Autodesk Fusion 360 part; units mm, degrees
(part 3 of 5)
  constraint tangent L16 A15
  constraint equal A14 A15
  constraint coincident A1.centre A6.centre
  constraint coincident P0 L19.end
  constraint coincident L19 A16.centre
  constraint equal A12 A16
  constraint coincident L12 A8.end
  constraint coincident L12 A17.centre
  constraint coincident A17.centre L21.start
  constraint perpendicular L12 L21
  constraint equal A12 A18
  constraint coincident L7 L22.end
  constraint perpendicular L7 L22
  constraint midpoint L20 L23.start
  constraint midpoint L18 L23.end
  constraint coincident L23 A19.centre
  constraint equal A12 A19
  constraint midpoint L13 L24.start
  constraint coincident L9 L24.end
  constraint perpendicular L13 L24
  constraint horizontal L25
  constraint perpendicular L25 L26
  constraint parallel L25 L27
  constraint parallel L26 L28
  constraint coincident L29 P9
  constraint coincident L30 P9
  constraint coincident P9 P8
  constraint horizontal L31
  constraint perpendicular L31 L32
  constraint parallel L31 L33
  constraint parallel L32 L34
  constraint coincident L35 P9
  constraint coincident L36 P9
  constraint coincident L32.end L33.start
  constraint coincident L33.end L34.start
  constraint coincident L31.start L34.end
  constraint concentric A29 A30
  constraint coincident L31.end L32.start
  constraint concentric A31 A32
  constraint equal A26 A28
  constraint equal A28 A30
  constraint equal A30 A31
  constraint equal A25 A29
  constraint equal A27 A29
  constraint equal A27 A32
  constraint midpoint A17 L21.end
  constraint coincident L12 L37.start
  constraint coincident L8 L37.end
  constraint perpendicular L8 L37
  constraint coincident L12 L38.start
  constraint coincident L8 L38.end
  constraint perpendicular L8 L38
  constraint coincident L4 L39.end
  constraint perpendicular L4 L39
  constraint perpendicular L0 L40
  constraint coincident L38 A33.end
  constraint coincident L12 A33.start
  constraint coincident L38.start L39.start
  constraint midpoint A33 L41.end
  constraint midpoint L41 A34.centre
  constraint coincident L38 A36.start
  constraint coincident L8 A36.end
  constraint coincident L38.end L40.start
  constraint midpoint A36 L42.end
  constraint midpoint L42 A37.centre
  constraint coincident L13 L43.end
  constraint perpendicular L13 L43
  constraint coincident L43 A39.start
  constraint coincident L13 A39.end
  constraint coincident L43.end A39.centre
  constraint midpoint A39 L44.end
  constraint midpoint L44 A40.centre
  constraint coincident L8 L45.end
  constraint perpendicular L8 L45
  constraint coincident L8 A42.start
  constraint coincident L8 A42.end
  constraint coincident L45.end A42.centre
  constraint midpoint A42 L46.start
  constraint coincident A37.centre A38.centre
  constraint coincident L46 L47.end
  constraint parallel L8 L47
  constraint coincident L47.end A43.centre
  constraint coincident A34.centre A35.centre
  constraint coincident L45 A18.centre
  constraint parallel L12 L48
  constraint coincident A18.centre A23.centre
  constraint coincident L12 L49.start
  constraint perpendicular L12 L49
  constraint coincident L8 L50.end
  constraint coincident L50 L51.start
  constraint coincident L37 L51.end
  constraint coincident L50 A45.start
  constraint coincident L12 A45.end
  constraint coincident L43 A45.end
  constraint coincident L49.start A45.centre
  constraint coincident L37 L52.end
  constraint midpoint A45 L53.end
  constraint midpoint L53 A46.centre
  constraint coincident L8 A48.start
  constraint coincident L50.end A48.centre
  constraint midpoint A48 L54.end
  constraint midpoint L54 A49.centre
  measures "d1_2" distance of P2 P3
  measures "d2_2" distance of L0 L4
  measures "d3_2" distance of P0 P1
  measures "d4_2" distance of P1 P2
  measures "d5_2" distance of P4 L6.end
  measures "d7_2" distance of P3 P4
  measures "d8_2" angle of L3 L4
  measures "d40_2" radius of A0
  measures "d47_2" radius of A10
  measures "d84_3" radius of A11
  measures "d85_2" diameter of A12
  measures "d88_2" radius of A9
  measures "d94_2" distance of L4.end A4.centre
  measures "d95_2" distance of A4.centre L12
  measures "d96_2" distance of L5.start A4.centre
  measures "d101_2" radius of A7
  measures "d102_2" radius of A2
  measures "d105_2" distance of A2.centre A13.centre
  measures "d111_2" distance of L17.start P6
  measures "d112_2" distance of A5.start P5
  measures "d113_2" radius of A14
  measures "d115_2" distance of A1.centre A16.centre
  measures "d120_2" radius of A17
  measures "d121_2" distance of A8.end A17.centre
  measures "d139_2" distance of L20 A19.centre
  measures "d153_2" distance of L23.end A19.centre
  measures "d234_2" distance of L26.end L27.end
  measures "d235_2" distance of L25.end L26.end
  measures "d236_2" distance of L32.end L33.end
  measures "d237_2" distance of L31.end L32.end
  measures "d238_2" diameter of A25
  measures "d240_2" distance of L24 P9
  measures "d392" distance of L13 L37
  measures "d393" distance of L37 L38
  measures "d448" distance of P9 L38
  measures "d465" radius of A33
  measures "d466" diameter of A34
  measures "d468" radius of A36
  measures "d469" diameter of A37
  measures "d478" radius of A39
  measures "d479" diameter of A40
  measures "d486" distance of L12 A34.centre
  measures "d487" distance of L38 A34.centre
  measures "d489" diameter of A43
  measures "d493" radius of A42
  measures "d508" distance of L37 L50
  measures "d510" radius of A45
  measures "d512" diameter of A46
  measures "d515" radius of A48
  measures "d516" diameter of A49
extrude "Extrude1'''''" add sketch "Base" along normal blind 60 separate body contours L0 L4 L7 A4 L8 L12 A9 L13 L22 L39 L40 L43 | L0 L1 L2 L3 L4 A0 A1 A2 A3 L8 A5 L9 A6 L10 A7 L11 A8 L12 L39 L40 | L5 L6 L7 A10 L22 | L8 L12 L37 L38 picked at (1.3333, -67.6667) picked at (115.3048, -1.3333) picked at (1.3333, -134) picked at (52.1667, -62.6667) makes body 5 in component "GM67 + printer"
sketch "Display cutout (2)" plane through (102.3013, 0, 177.191) normal (-0.5, 0, -0.866025) x (0, -1, 0) in component "GM67 + printer"
  line L0 (0, -151.0474) -> (0, -81.0474)
  line L1 (-60, -81.0474) -> (-60, -151.0474)
  line L2 (0, -116.0474) -> (-60, -116.0474) construction
  line L3 (0, -81.0474) -> (-60, -81.0474)
  line L4 (-60, -151.0474) -> (0, -151.0474)
  line L5 (-21.675, -129.0474) -> (-21.675, -123.5474)
  line L6 (-16.175, -108.5474) -> (-16.175, -99.5474)
  line L7 (-16.175, -129.0474) -> (-43.825, -129.0474)
  line L8 (-16.175, -99.5474) -> (-16.175, -104.2474)
  line L9 (-16.175, -99.5474) -> (-43.825, -99.5474)
  line L10 (-21.675, -99.5474) -> (-16.175, -99.5474)
  line L11 (-16.175, -104.2474) -> (-21.675, -104.2474)
  line L12 (-21.675, -104.2474) -> (-21.675, -99.5474)
  line L13 (-16.175, -123.5474) -> (-16.175, -129.0474)
  line L14 (-16.175, -123.5474) -> (-16.175, -108.5474)
  line L15 (-43.825, -108.5474) -> (-43.825, -123.5474)
  line L16 (-38.325, -99.5474) -> (-38.325, -104.2474)
  line L17 (-16.175, -108.5474) -> (-43.825, -123.5474) construction
  line L18 (-43.825, -129.0474) -> (-43.825, -123.5474)
  line L19 (-43.825, -99.5474) -> (-43.825, -108.5474)
  line L20 (-38.325, -104.2474) -> (-43.825, -104.2474)
  line L21 (-43.825, -104.2474) -> (-43.825, -99.5474)
  line L22 (-43.825, -123.5474) -> (-16.175, -123.5474)
  line L23 (-43.825, -108.5474) -> (-16.175, -108.5474)
  line L24 (-16.175, -108.5474) -> (-43.825, -108.5474)
  line L25 (-43.825, -123.5474) -> (-16.175, -123.5474)
  line L26 (-38.325, -129.0474) -> (-38.325, -123.5474)
  line L27 (-43.825, -108.5474) -> (-16.175, -123.5474) construction
  line L28 (-43.825, -99.5474) -> (-38.325, -99.5474)
  line L29 (-13.675, -131.5474) -> (-46.325, -131.5474) construction
  line L30 (-46.325, -131.5474) -> (-46.325, -97.0474) construction
  line L31 (-46.325, -97.0474) -> (-13.675, -97.0474) construction
  line L32 (-13.675, -97.0474) -> (-13.675, -131.5474) construction
  circle A0 centre (-46.325, -131.5474) radius 0.95
  circle A1 centre (-13.675, -131.5474) radius 0.95
  circle A2 centre (-46.325, -97.0474) radius 0.95
  circle A3 centre (-13.675, -97.0474) radius 0.95
  line L33 (-17.675, -123.5474) -> (-17.675, -108.5474)
  line L34 (-42.325, -123.5474) -> (-42.325, -108.5474)
  point P0 (-30, -116.0474)
  point P1 (-30, -116.0474)
  point P2 (-30, -116.0474)
  point P3 (0, -117.3108)
  dimension "d64_2" = 27.65
  dimension "d65_2" = 15
  dimension "d66_2" = 5.5
  dimension "d67_2" = 9
  dimension "d68_2" = 5.5
  dimension "d69_2" = 5.5
  dimension "d70_2" = 4.7
  dimension "d225_2" = 29.5
  dimension "d226_2" = 24.8
  dimension "d645" = 30
  dimension "d646" = 30
  dimension "d647" = 2.5
  dimension "d648" = 2.5
  dimension "d649" = 2.5
  dimension "d650" = 2.5
  dimension "d651" = 35
  dimension "d652" = 1.9
  dimension "d658" = 1.5
  dimension "d659" = 1.5
  constraint midpoint L0 L2.start
  constraint midpoint L1 L2.end
  constraint perpendicular L15 L24
  constraint parallel L24 L25
  constraint parallel L14 L15
  constraint coincident P2 L17
  constraint coincident P2 L27
  constraint perpendicular L13 L22
  constraint parallel L7 L22
  constraint parallel L13 L18
  constraint perpendicular L6 L23
  constraint parallel L9 L23
  constraint parallel L6 L19
  constraint coincident L26.start L7
  constraint coincident L26.end L25
  constraint perpendicular L25 L26
  constraint coincident L5.start L7
  constraint coincident L5.end L22
  constraint perpendicular L5 L22
  constraint collinear L16 L26
  constraint coincident L8.end L6
  constraint coincident L10.start L9
  constraint collinear L5 L12
  constraint collinear L11 L20
  constraint coincident P2 P1
  constraint midpoint L2 P2
  constraint horizontal L29
  constraint vertical L30
  constraint horizontal L31
  constraint vertical L32
  constraint coincident L29.end L30.start
  constraint coincident L29.start L32.end
  constraint coincident L30.end L31.start
  constraint coincident L31.end L32.start
  constraint equal A0 A1
  constraint equal A0 A2
  constraint equal A2 A3
  constraint coincident L22 L33.start
  constraint coincident L24 L33.end
  constraint perpendicular L24 L33
  constraint coincident L22 L34.start
  constraint coincident L23 L34.end
  constraint perpendicular L23 L34
  measures "d64_2" distance of L15.end L13.start
  measures "d65_2" distance of L15.end L15.start
  measures "d66_2" distance of L15.end L7.end
  measures "d67_2" distance of L15.start L9.end
  measures "d68_2" distance of L18 L26
  measures "d69_2" distance of L5 L13
  measures "d70_2" distance of L20 L28
  measures "d225_2" distance of L7 L9
  measures "d226_2" distance of L7 L20
  measures "d645" horizontal distance of P2 P3
  measures "d646" distance of L1 P2
  measures "d647" distance of L15 L30
  measures "d648" distance of L14 L32
  measures "d649" distance of L7 L29
  measures "d650" distance of L9 L31
  measures "d651" distance of L4 P2
  measures "d652" diameter of A1
  measures "d658" distance of L14 L33
  measures "d659" distance of L15 L34
extrude "Extrude8''" add sketch "Base" against normal blind 4 contours L0 L4 L7 A4 L8 L12 A9 L13 L22 L39 L40 L43 | L0 L1 L2 L3 L4 A0 A1 A2 A3 L8 A5 L9 A6 L10 A7 L11 A8 L12 L39 L40 | L5 L6 L7 A10 L22 | L8 L12 L37 L38 | L8 L38 A36 | L8 L37 L51 A48 | L8 L9 L10 L11 A8 L12 S0 L16 L17 L18 A14 A15 S1 A17 L38 A33 A36 A42 | L8 L12 L13 A11 L37 L43 A39 L51 A45 L52 A48 | L8 A42 | L12 L38 A33 | L8 L13 A11 | L12 L37 L43 A45 L52 | L8 A5 L16 L17 L18 A14 A15 | L12 A17 | L13 L43 A39 | A9 L13 L43 | A6 S1 | A7 S0 | A12 | A13 | A16 | A18 | A19 | A20 | A21 | A22 | A23 | A24 | L25 L28 A30 | L25 L28 A30 | L25 L31 A30 A31 | L26 L27 L28 L31 A26 A28 A30 A31 | L25 L26 A31 | L25 L26 A31 | L27 L28 A28 | L27 L28 A28 | L26 L27 A26 | L26 L27 A26 | A25 | A27 | A29 | A32 | A34 | A35 | A37 | A38 | A40 | A41 | A43 | A44 | A46 | A47 | A49 | A50 | L55 L56 L57 S2 S3 L58 L59 L60 L61 | S4 S5 S6 S7 S8 S9 S10 S11 S12 S13 S14 S15 S16 S17 L62 S18 S19 S20 S21 S22 S23 S24 L63 S25 S26 L64 S27 | S28 S29 S30 S31 S32 S33 S34 S35 S36 L65 | L66 L67 L68 S37 S38 S39 S40 S41 L69 L70 L71 S42 S43 S44 S45 S46 L72 L73 | L74 L75 L76 L77 L78 L79 L80 L81 L82 L83 L84 L85 | L86 S47 S48 S49 S50 S51 S52 S53 S54 S55 L87 S56 S57 S58 S59 | L88 S60 S61 S62 S63 | L89 L90 L91 S64 S65 S66 S67 S68 S69 S70 L92 L93 L94 S71 S72 S73 S74 S75 L95 L96 L97 S76 S77 S78 S79 S80 L98 L99 | L100 S81 S82 S83 S84 S85 S86 S87 S88 S89 L101 S90 S91 S92 S93 | L102 S94 S95 S96 S97 | L103 L104 L105 S98 S99 S100 L106 S101 S102 S103 S104 L107 L108 | L109 S105 S106 S107 S108 L110 L111 L112 L113 L114 L115 L116 L117 L118 L119 L120 S109 S110 S111 S112 | L121 L122 L123 L124 L125 L126 L127 L128 L129 L130 L131 L132 | S113 S114 S115 S116 S117 S118 S119 S120 S121 | S122 S123 S124 S125 S126 S127 S128 S129 | L133 L134 L135 S130 S131 S132 S133 S134 S135 S136 L136 L137 L138 S137 S138 S139 S140 S141 L139 L140 L141 S142 S143 S144 S145 S146 L142 L143 | L144 S147 S148 S149 S150 S151 S152 S153 S154 S155 L145 S156 S157 S158 S159 | L146 S160 S161 S162 S163 | L147 L148 L149 L150 L151 L152 L153 L154 | L155 L156 S164 S165 L157 | L158 S166 S167 S168 S169 S170 L159 L160 L161 S171 S172 S173 S174 S175 S176 L162 L163 L164 L165 | L166 S177 S178 S179 S180 L167 L168 L169 L170 L171 L172 L173 L174 L175 L176 L177 S181 S182 S183 S184 | S185 S186 S187 S188 S189 S190 S191 S192 S193 | S194 S195 S196 S197 S198 S199 S200 S201 | L178 L179 L180 S202 S203 S204 S205 S206 S207 S208 L181 L182 L183 S209 S210 S211 S212 S213 L184 L185 L186 S214 S215 S216 S217 S218 L187 L188 | S219 S220 S221 S222 S223 S224 S225 S226 S227 S228 S229 S230 S231 S232 L189 S233 S234 S235 S236 S237 S238 S239 L190 S240 S241 L191 S242 | S243 S244 S245 S246 S247 S248 S249 S250 S251 L192 | L193 S252 S253 S254 S255 L194 L195 L196 L197 L198 L199 L200 L201 L202 L203 L204 S256 S257 S258 S259 | L205 L206 L207 L208 | L209 L210 L211 L212 | S260 S261 S262 S263 S264 S265 S266 S267 S268 | S269 S270 S271 S272 S273 S274 S275 S276 | L213 L214 L215 S277 S278 S279 S280 S281 L216 L217 L218 S282 S283 S284 S285 S286 L219 L220 picked at (1.3333, -67.6667) picked at (115.3048, -1.3333) picked at (1.3333, -134) picked at (52.1667, -62.6667) picked at (54.3547, -10.8354) picked at (48.6321, -7.7213) picked at (194.8489, -92.1347) picked at (19.6078, -37.0924) picked at (111.3605, -5.0148) picked at (54.3547, -89.1646) picked at (4.8547, -10.8354) picked at (48.6321, -92.2787) picked at (189.6849, -9.3579) picked at (111.3605, -94.9852) picked at (4.8547, -89.1646) picked at (8.5199, -96.8371) picked at (232.0947, -97.7086) picked at (161.4527, -131.5761) picked at (5.8446, -6.4517) picked at (165.8157, -135.0059) picked at (235.0107, -95.0561) picked at (116.851, -93.8237) picked at (185.7147, -8.8468) picked at (8.9867, -6.9402) picked at (187.9895, -7.222) picked at (232.2154, -94.0645) picked at (118.8458, -94.7215) picked at (163.0278, -133.6914) picked at (134.6465, -19.4866) picked at (131.9015, -17.0378) picked at (94.8167, -18.8853) picked at (112.5824, -57.6314) picked at (72.3535, -19.4866) picked at (75.1014, -17.0408) picked at (131.9015, -80.3003) picked at (134.6465, -77.8515) picked at (72.3535, -77.8515) picked at (71.8718, -77.0676) picked at (74.2427, -77.8131) picked at (132.8417, -78.8001) picked at (132.7147, -19.0317) picked at (73.9155, -18.9537) picked at (56.9587, -93.6573) picked at (56.0557, -91.0277) picked at (55.1805, -6.2756) picked at (54.8223, -5.2785) picked at (7.3535, -92.2324) picked at (6.5557, -95.3155) picked at (116.5543, -7.2819) picked at (115.2444, -6.2991) picked at (45.3018, -93.6573) picked at (44.3988, -91.0277) picked at (43.5237, -6.2756) picked at (43.1655, -5.2785) picked at (204.0655, -50.3607) picked at (198.4166, -49.6797) picked at (199.482, -49.9612) picked at (197.0464, -50.5358) picked at (187.6251, -51.1213) picked at (184.3656, -50.4915) picked at (184.9086, -51.4476) picked at (182.292, -50.5028) picked at (174.6623, -50.4915) picked at (175.2053, -51.4476) picked at (172.5955, -50.5085) picked at (169.9477, -50.413) picked at (204.3088, -43.3178) picked at (196.6385, -42.5157) picked at (198.0941, -41.6416) picked at (195.4945, -42.6993) picked at (187.8649, -42.6879) picked at (188.4079, -43.6441) picked at (181.4279, -43.2166) picked at (182.5125, -43.3803) picked at (177.0634, -42.6334) picked at (175.3774, -42.6095) picked at (171.0109, -42.5157) picked at (172.4665, -41.6416) picked at (169.867, -42.6993) picked at (161.5339, -41.8761) picked at (162.5994, -42.1577) picked at (159.8488, -42.6095) picked at (158.015, -45.3948) picked at (158.015, -42.0729) picked at (153.9304, -42.5157) picked at (155.386, -41.6416) picked at (152.7865, -42.7323) bodies 5 in component "GM67 + printer"
sketch "Sensor cutout (2)" plane through (0, 0, 96) normal (0, 0, -1) x (1, 0, 0) in component "GM67 + printer"
  line L0 (125.3397, 0) -> (53.5, 0)
  line L1 (19, 0) -> (19, -60)
  line L2 (53.5, -60) -> (125.3397, -60)
  line L3 (125.3397, -60) -> (125.3397, 0)
  line L4 (19, -30) -> (125.3397, -30) construction
  circle A0 centre (69, -30) radius 13
  line L5 (53.5, 0) -> (53.5, -60)
  line L6 (49.5, 0) -> (19, 0)
  line L7 (19, -60) -> (49.5, -60)
  line L8 (49.5, -60) -> (49.5, 0)
  dimension "d48_2" = 26
  dimension "d49_2" = 50
  constraint midpoint L1 L4.start
  constraint coincident L4 A0.centre
  measures "d48_2" diameter of A0
  measures "d49_2" distance of L4.start A0.centre
sketch "Power cutout (2)" plane through (0, 0, 4) normal (0, 0, 1) x (-1, 0, 0) in component "GM67 + printer"
  line L0 (-53.5, 0) -> (-183.0748, 0)
  line L1 (-183.0748, 0) -> (-183.0748, -60)
  line L2 (-183.0748, -60) -> (-53.5, -60)
  line L3 (-4, -60) -> (-4, 0)
  line L4 (-4, -30) -> (-183.0748, -30) construction
  circle A0 centre (-24, -30) radius 6.3
  line L5 (-102.7993, -29.1827) -> (-102.7993, -29)
  line L6 (-53.5, -60) -> (-53.5, 0)
  line L7 (-4, 0) -> (-49.5, 0)
  line L8 (-49.5, 0) -> (-49.5, -60)
  line L9 (-49.5, -60) -> (-4, -60)
  line L10 (-32.55, -34.9363) -> (-24, -39.8727)
  line L11 (-24, -39.8727) -> (-15.45, -34.9363)
  line L12 (-15.45, -34.9363) -> (-15.45, -25.0637)
  line L13 (-15.45, -25.0637) -> (-24, -20.1273)
  line L14 (-24, -20.1273) -> (-32.55, -25.0637)
  line L15 (-32.55, -25.0637) -> (-32.55, -34.9363)
  point P0 (-24, -30)
  point P1 (-24, -30)
  dimension "d52_2" = 12.6
  dimension "d53_2" = 20
  dimension "d432" = 8.55
  constraint midpoint L3 L4.start
  constraint midpoint L1 L4.end
  constraint coincident L4 P1
  constraint coincident P1 P0
  measures "d52_2" diameter of A0
  measures "d53_2" distance of L3 P1
  measures "d432" distance of P1 L15
extrude "Extrude3'''" cut sketch "Display cutout (2)" against normal up to surface (4 mm away) contours L22 L23 L24 L25 L33 L34 | L14 L22 L23 L24 L25 L33 | L15 L22 L23 L24 L25 L34 picked at (-32.775, -113.5474) picked at (-16.675, -118.5474) picked at (-42.825, -118.5474) bodies 5 in component "GM67 + printer"
extrude "Extrude4'" cut sketch "Display cutout (2)" against normal blind 1.1 contours L5 L7 L13 L22 L25 | L7 L18 L22 L25 L26 | L6 L8 L9 L10 L11 L12 | L9 L16 L19 L20 L21 L28 picked at (-18.5083, -127.2141) picked at (-41.4917, -127.2141) picked at (-18.0083, -101.1141) picked at (-41.9917, -102.6807) bodies 5 in component "GM67 + printer"
extrude "Extrude5'" cut sketch "Display cutout (2)" against normal blind 2.5 contours L5 L7 L22 L25 L26 | L14 L22 L23 L24 L25 L33 | L15 L22 L23 L24 L25 L34 | L6 L9 L11 L12 L16 L19 L20 L23 L24 picked at (-32.775, -125.3807) picked at (-16.675, -118.5474) picked at (-42.825, -118.5474) picked at (-27.225, -107.1141) bodies 5 in component "GM67 + printer"
extrude "Extrude12'" [suppressed] in component "GM67 + printer"
sketch "Button cutout (2)" plane through (140.3372, 0, -81.0237) normal (-0.866025, 0, 0.5) x (0, -1, 0) in component "GM67 + printer"
  line L0 (0, 104.5278) -> (0, 193.6025)
  line L1 (0, 193.6025) -> (-60, 193.6025)
  line L2 (-60, 193.6025) -> (-60, 104.5278)
  line L3 (-60, 104.5278) -> (0, 104.5278)
  line L4 (-64, 123.2917) -> (-64, 136.282)
  line L5 (-64, 136.282) -> (-64, 152.6218)
  line L6 (-64, 167.6218) -> (-64, 152.6218)
  line L7 (-64, 70.1218) -> (-64, 123.2917)
  line L8 (0, 149.0652) -> (-64, 149.0652) construction
  line L9 (-32, 149.0652) -> (-32, 191.1025) construction
  circle A0 centre (-48, 149.0652) radius 6.25
  circle A1 centre (-16, 149.0652) radius 6.25
  circle A2 centre (-48, 149.0652) radius 8 construction
  circle A3 centre (-16, 149.0652) radius 8 construction
  dimension "d228_2" = 12.5
  dimension "d229_2" = 16
  dimension "d230_2" = 32
  dimension "d233_2" = 16
  constraint midpoint L0 L8.start
  constraint coincident L4 L8.end
  constraint perpendicular L4 L8
  constraint midpoint L8 L9.start
  constraint coincident L8 A0.centre
  constraint symmetric L9 A0 A1
  constraint concentric A0 A2
  constraint symmetric L9 A2 A3
  measures "d228_2" diameter of A0
  measures "d229_2" distance of L7 A0.centre
  measures "d230_2" distance of A0.centre A1.centre
  measures "d233_2" diameter of A2
extrude "Extrude21'" cut sketch "Button cutout (2)" against normal up to surface (4 mm away) contours A0 | A1 picked at (-46.0092, 149.0582) picked at (-17.5272, 151.7103) bodies 5 in component "GM67 + printer"
extrude "Extrude22'" add sketch "Base" along normal blind 3 contours L25 L28 A30 | L25 L28 A30 | L25 L26 A31 | L25 L26 A31 | L27 L28 A28 | L27 L28 A28 | L26 L27 A26 | L26 L27 A26 picked at (134.6465, -19.4866) picked at (131.9015, -17.0378) picked at (72.3535, -19.4866) picked at (75.1014, -17.0408) picked at (131.9015, -80.3003) picked at (134.6465, -77.8515) picked at (72.3535, -77.8515) picked at (71.8718, -77.0676) bodies 5 in component "GM67 + printer"
fillet "Fillet6'" radius 1.5 4 edges at (129.7835, 0, 76.9215) (70.7835, 0, 76.9215) (129.7835, 0, 17.9215) (70.7835, 0, 17.9215) on bodies 5 in component "GM67 + printer"
extrude "Extrude23'" cut 4 faces at (132.8417, 0, 78.8001) (74.2427, 0, 77.8131) (132.7147, 0, 19.3064) (73.9155, 0, 18.9537) along direction (0, -1, 0) blind 2 on bodies 5 bodies 5 in component "GM67 + printer"
extrude "Extrude1''''''" add sketch "Sketch1 (5)" against normal blind 4 separate body contours L6 L7 L8 L9 | L6 L13 L14 L15 | L8 L10 L11 L12 picked at (-12.25, 43.4167) picked at (15.5833, 48.0833) picked at (-15.5833, -48.0833) makes body 6 in component "Trial printer"
extrude "Extrude2''''" add sketch "Sketch1 (5)" along normal blind 45.5 contours L6 L13 L14 L15 | L8 L10 L11 L12 picked at (15.5833, 48.0833) picked at (-15.5833, -48.0833) bodies 6 in component "Trial printer"
sketch "Sketch2 (2)" plane through (0, 45.5, 0) normal (0, 1, 0) x (-1, 0, 0) in component "Trial printer"
  line L0 (46.75, 46.75) -> (46.75, 50.75)
  line L1 (46.75, 50.75) -> (-46.75, 50.75)
  line L2 (-46.75, 50.75) -> (-46.75, 46.75)
  line L3 (-46.75, 46.75) -> (46.75, 46.75)
  line L4 (-46.75, 50.75) -> (46.75, 50.75)
  line L5 (46.75, 50.75) -> (46.75, -50.75)
  line L6 (46.75, -50.75) -> (-46.75, -50.75)
  line L7 (-46.75, -50.75) -> (-46.75, 50.75)
  line L8 (46.75, 29.25) -> (-46.75, 29.25) construction
  circle A0 centre (25, 29.25) radius 3.5
  circle A1 centre (25, 29.25) radius 7.5
  circle A2 centre (25, 29.25) radius 1.75
  line L9 (0, 50.75) -> (0, -51.9724) construction
  circle A3 centre (-25, 29.25) radius 7.5
  circle A4 centre (-25, 29.25) radius 3.5
  circle A5 centre (-25, 29.25) radius 1.75
  line L10 (36.75, 36.75) -> (-36.75, 36.75)
  point P0 (46.75, 50.75)
  point P1 (-46.75, 50.75)
  point P2 (-46.75, -50.75)
  point P3 (46.75, -50.75)
  dimension "d371" = 25
  dimension "d372" = 7
  dimension "d373" = 3.5
  dimension "d374" = 15
  dimension "d389" = 7.5
  constraint coincident P1 L1.end
  constraint coincident P0 L0.end
  constraint coincident P3 L5.end
  constraint coincident P2 L6.end
  constraint coincident L5 L8.start
  constraint coincident L7 L8.end
  constraint perpendicular L7 L8
  constraint coincident L8 A0.centre
  constraint concentric A0 A1
  constraint concentric A0 A2
  constraint midpoint L4 L9.start
  constraint perpendicular L6 L9
  constraint symmetric A0 L9 A4
  constraint symmetric A1 L9 A3
  constraint symmetric A2 L9 A5
  measures "d371" horizontal distance of origin A0.centre
  measures "d372" diameter of A0
  measures "d373" diameter of A2
  measures "d374" diameter of A1
  measures "d389" distance of A0.centre L10
extrude "Extrude3''''" add sketch "Sketch2 (2)" along normal blind 4 contours L0 L1 L2 L3 L4 L5 L7 | L3 L5 L6 L7 | A0 | A1 | A2 | A3 | A4 | A5 picked at (15.5833, 48.0833) picked at (-7.3766, -26.393) picked at (27.8971, 28.9892) picked at (24.546, 35.3863) picked at (24.3796, 29.7448) picked at (-25.454, 35.3863) picked at (-22.1029, 28.9892) picked at (-25.6204, 29.7448) bodies 6 in component "Trial printer"
extrude "Extrude4''" add sketch "Sketch2 (2)" against normal blind 15 contours A0 | A4 picked at (27.8971, 28.9892) picked at (-22.1029, 28.9892) bodies 6 in component "Trial printer"
extrude "Extrude5''" add sketch "Sketch2 (2)" against normal blind 15 contours A1 | A3 picked at (24.546, 35.3863) picked at (-25.454, 35.3863) bodies 6 in component "Trial printer"
extrude "Extrude6'" cut sketch "Sketch2 (2)" against normal blind 4 from surface at 4 contours A0 | A2 | A4 | A5 picked at (27.8971, 28.9892) picked at (24.3796, 29.7448) picked at (-22.1029, 28.9892) picked at (-25.6204, 29.7448) bodies 6 in component "Trial printer"
fillet "Fillet1'" radius 6 2 edges at (0, 0, 46.75) (0, 0, -46.75) on bodies 6 in component "Trial printer"
fillet "Fillet2" radius 10 2 edges at (0, -4, -50.75) (0, -4, 50.75) on bodies 6 in component "Trial printer"
fillet "Fillet3" radius 10 2 edges at (-18.0075, 45.5, 26.5379) (31.9925, 45.5, 26.5379) on bodies 6 in component "Trial printer"
sketch "Printer extrusion" plane through (0, 60, 0) normal (0, 1, 0) x (-1, 0, 0) in component "GM67 + printer"
  line L0 (-49.5, 96) -> (-19, 96)
  arc A0 (-19, 96) -> (-4, 103.3381) centre (-19, 115) ccw
  line L1 (-4, 103.3381) -> (-4, 4)
  line L2 (-4, 4) -> (-49.5, 4)
  line L3 (-49.5, 4) -> (-49.5, 96)
  arc A1 (-157.4641, 132.641) -> (-172.4904, 136.6673) centre (-166.9904, 127.141) ccw
  line L4 (-157.4641, 132.641) -> (-141.7942, 105.5)
  arc A2 (-141.7942, 105.5) -> (-125.3397, 96) centre (-125.3397, 115) ccw
  line L5 (-125.3397, 96) -> (-53.5, 96)
  line L6 (-53.5, 96) -> (-53.5, 4)
  line L7 (-53.5, 4) -> (-183.0748, 4)
  arc A3 (-192.6011, 9.5) -> (-183.0748, 4) centre (-183.0748, 15) ccw
  line L8 (-192.6011, 9.5) -> (-237.1384, 86.641)
  arc A4 (-233.1122, 101.6673) -> (-237.1384, 86.641) centre (-227.6122, 92.141) ccw
  line L9 (-233.1122, 101.6673) -> (-172.4904, 136.6673)
  line L10 (0, 145) -> (-1, 145)
  arc A5 (-1, 145) -> (-4, 142) centre (-1, 142) ccw
  line L11 (-4, 142) -> (-4, 115)
  arc A6 (-19, 100) -> (-4, 115) centre (-19, 115) ccw
  line L12 (-19, 100) -> (-125.3397, 100)
  arc A7 (-138.3301, 107.5) -> (-125.3397, 100) centre (-125.3397, 115) ccw
  line L13 (-138.3301, 107.5) -> (-154, 134.641)
  arc A8 (-154, 134.641) -> (-174.4904, 140.1314) centre (-166.9904, 127.141) ccw
  line L14 (-174.4904, 140.1314) -> (-235.1122, 105.1314)
  arc A9 (-235.1122, 105.1314) -> (-240.6025, 84.641) centre (-227.6122, 92.141) ccw
  line L15 (-240.6025, 84.641) -> (-196.0652, 7.5)
  arc A10 (-196.0652, 7.5) -> (-183.0748, 0) centre (-183.0748, 15) ccw
  line L16 (-183.0748, 0) -> (0, 0)
  line L17 (0, 0) -> (0, 145)
  arc A11 (-1, 145) -> (-4, 142) centre (-1, 142) ccw
  line L18 (-4, 115) -> (-4, 142)
  arc A12 (-19, 100) -> (-4, 115) centre (-19, 115) ccw
  line L19 (0, 145) -> (0, 0)
  line L20 (-49.5, 96) -> (-49.5, 4)
  arc A13 (-19, 96) -> (-4, 103.3381) centre (-19, 115) ccw
  line L21 (-4, 103.3381) -> (-4, 4)
  line L22 (-53.5, 100) -> (-19, 100)
  line L23 (-49.5, 96) -> (-19, 96)
  line L24 (-53.5, 0) -> (0, 0)
  line L25 (-49.5, 4) -> (-4, 4)
  line L26 (-53.5, 100) -> (-53.5, 0)
  point P0 (0, 145)
  constraint coincident A6.start L12.start
  constraint coincident L0.start L3.end
  constraint coincident L0.end A0.start
  constraint coincident L16.end L17.start
  constraint coincident L2.end L3.start
  constraint coincident L1.end L2.start
  constraint perpendicular L24 L26
extrude "Extrude24" add sketch "Printer extrusion" along normal blind 93.5 contours L6 L10 A5 L11 A6 L12 L16 L17 A11 L18 A12 L19 L22 L24 L26 picked at (-1.3333, 82.7794) bodies 5 in component "GM67 + printer"
sketch "Printer Powersupply cutout" plane through (53.5, 0, 0) normal (1, 0, 0) x (0, 1, 0) in component "GM67 + printer"
  line L0 (0, 96) -> (0, 4)
  line L1 (0, 4) -> (60, 4)
  line L2 (60, 4) -> (60, 0)
  line L3 (60, 0) -> (153.5, 0)
  line L4 (153.5, 0) -> (153.5, 100)
  line L5 (153.5, 100) -> (60, 100)
  line L6 (60, 100) -> (60, 96)
  line L7 (60, 96) -> (0, 96)
  line L8 (64, 0) -> (64, 100) construction
  line L9 (153.5, 100) -> (64, 0) construction
  line L10 (153.5, 0) -> (64, 100) construction
  line L11 (145.5, 86.75) -> (72, 86.75)
  line L12 (72, 86.75) -> (72, 13.25)
  line L13 (72, 13.25) -> (145.5, 13.25)
  line L14 (145.5, 13.25) -> (145.5, 86.75)
  line L15 (145.5, 86.75) -> (72, 13.25) construction
  line L16 (72, 86.75) -> (145.5, 13.25) construction
  line L17 (30, 4) -> (30, 96) construction
  circle A0 centre (30, 39.75) radius 1.75
  circle A1 centre (30, 78.85) radius 1.75
  line L18 (4.5, 93.5) -> (55.5, 93.5) construction
  line L19 (55.5, 93.5) -> (55.5, 31) construction
  line L20 (55.5, 31) -> (4.5, 31) construction
  line L21 (4.5, 31) -> (4.5, 93.5) construction
  line L22 (4.5, 93.5) -> (55.5, 31) construction
  line L23 (55.5, 93.5) -> (4.5, 31) construction
  line L24 (40, 39.75) -> (40, 78.85)
  arc A2 (40, 78.85) -> (20, 78.85) centre (30, 78.85) ccw
  line L25 (20, 78.85) -> (20, 39.75)
  arc A3 (20, 39.75) -> (40, 39.75) centre (30, 39.75) ccw
  line L26 (30, 39.75) -> (30, 78.85) construction
  line L27 (15.5, 18) -> (15.5, 31) construction
  line L28 (55.5, 31) -> (55.5, 18) construction
  line L29 (55.5, 18) -> (15.5, 18) construction
  line L30 (0, 17.5) -> (64, 17.5) construction
  line L31 (14, 17.5) -> (46, 17.5) construction
  line L32 (0, 4) -> (60, 4)
  line L33 (15.5, 17.5) -> (55.5, 17.5) construction
  circle A4 centre (30, 78.85) radius 3
  circle A5 centre (30, 39.75) radius 3
  line L34 (145.5, 20.75) -> (72, 20.75) construction
  line L35 (108.75, 86.75) -> (108.75, 13.25) construction
  circle A6 centre (133.75, 20.75) radius 1.75
  circle A7 centre (133.75, 20.75) radius 6
  circle A8 centre (83.75, 20.75) radius 6
  circle A9 centre (83.75, 20.75) radius 1.75
  circle A10 centre (133.75, 20.75) radius 3.5
  circle A11 centre (83.75, 20.75) radius 3.5
  line L36 (60.4248, 4) -> (60, 96) construction
  line L37 (50, 21) -> (10, 21)
  arc A12 (10, 21) -> (10, 14) centre (10, 17.5) ccw
  line L38 (10, 14) -> (50, 14)
  arc A13 (50, 14) -> (50, 21) centre (50, 17.5) ccw
  line L39 (50, 17.5) -> (10, 17.5) construction
  point P0 (106.75, 50)
  point P1 (108.75, 50)
  point P2 (30, 62.25)
  point P3 (30, 17.5)
  point P4 (30, 17.5)
  dimension "d401" = 4
  dimension "d402" = 73.5
  dimension "d403" = 73.5
  dimension "d409" = 64
  dimension "d410" = 92
  dimension "d411" = 39.1
  dimension "d412" = 3.5
  dimension "d413" = 3.5
  dimension "d414" = 51
  dimension "d415" = 62.5
  dimension "d418" = 20
  dimension "d423" = 14.65
  dimension "d424" = 2.5
  dimension "d430" = 13
  dimension "d431" = 40
  dimension "d438" = 13.5
  dimension "d439" = 16
  dimension "d449" = 6
  dimension "d452" = 7.5
  dimension "d453" = 25
  dimension "d454" = 3.5
  dimension "d455" = 12
  dimension "d456" = 7
  dimension "d609" = 20
  dimension "d610" = 3.5
  constraint coincident L3 L8.start
  constraint coincident L5 L8.end
  constraint perpendicular L5 L8
  constraint coincident L4.end L5.start
  constraint coincident L3.end L4.start
  constraint horizontal L11
  constraint perpendicular L11 L12
  constraint parallel L11 L13
  constraint parallel L12 L14
  constraint coincident L15 P1
  constraint coincident L16 P1
  constraint midpoint L9 P1
  constraint midpoint L1 L17.start
  constraint midpoint L7 L17.end
  constraint coincident L17 A0.centre
  constraint coincident L17 A1.centre
  constraint horizontal L18
  constraint perpendicular L18 L19
  constraint parallel L18 L20
  constraint parallel L19 L21
  constraint coincident L22 P2
  constraint coincident L23 P2
  constraint coincident L17 P2
  constraint tangent L24 A2
  constraint tangent A2 L25
  constraint parallel L24 L25
  constraint tangent L25 A3
  constraint tangent L24 A3
  constraint coincident A1.centre A2.centre
  constraint parallel L17 L26
  constraint coincident A0.centre A3.centre
  constraint coincident L20 L27.end
  constraint perpendicular L20 L27
  constraint perpendicular L20 L28
  constraint perpendicular L27 L29
  constraint coincident L0 L30.start
  constraint coincident L8 L30.end
  constraint perpendicular L8 L30
  constraint coincident L30 L31.end
  constraint perpendicular L17 L31
  constraint coincident L17 P4
  constraint midpoint L31 P4
  constraint coincident L30 L33.end
  constraint perpendicular L28 L33
  constraint coincident L27 L33.start
  constraint coincident L28 L33.end
  constraint concentric A1 A4
  constraint concentric A0 A5
  constraint equal A4 A5
  constraint coincident L14 L34.start
  constraint coincident L12 L34.end
  constraint perpendicular L12 L34
  constraint midpoint L11 L35.start
  constraint midpoint L13 L35.end
  constraint coincident L34 A6.centre
  constraint concentric A6 A7
  constraint symmetric L35 A6 A9
  constraint symmetric L35 A7 A8
  constraint concentric A6 A10
  constraint symmetric L35 A10 A11
  constraint coincident L6.end L7.start
  constraint tangent L37 A12
  constraint tangent A12 L38
  constraint parallel L37 L38
  constraint tangent L38 A13
  constraint tangent L37 A13
  constraint coincident L30 A12.centre
  constraint parallel L30 L39
  constraint coincident P4 P3
  constraint midpoint L39 P4
  measures "d401" distance of L2.end L8.start
  measures "d402" distance of L12.end L13.end
  measures "d403" distance of L11.end L12.end
  measures "d409" distance of L0 L8
  measures "d410" distance of L1 L7
  measures "d411" distance of A0.centre A1.centre
  measures "d412" diameter of A0
  measures "d413" diameter of A1
  measures "d414" distance of L19.end L20.end
  measures "d415" distance of L18.end L19.end
  measures "d418" diameter of A2
  measures "d423" distance of L18 A1.centre
  measures "d424" distance of L7 L18
  measures "d430" distance of L19.end L28.end
  measures "d431" distance of L27.start L28.end
  measures "d438" distance of L30 L32
  measures "d439" distance of L31.end P4
  measures "d449" diameter of A5
  measures "d452" distance of L13 L34
  measures "d453" horizontal distance of P1 A6.centre
  measures "d454" diameter of A6
  measures "d455" diameter of A7
  measures "d456" diameter of A10
  measures "d609" distance of A12.centre P4
  measures "d610" distance of L38 P4
extrude "Extrude25" cut sketch "Printer Powersupply cutout" against normal up to surface (4 mm away) contours L11 L12 L13 L14 | A6 | A7 | A8 | A9 | A10 | A11 picked at (116.0833, 66.4821) picked at (133.1154, 21.2809) picked at (135.352, 15.8524) picked at (88.8813, 20.278) picked at (84.1137, 21.38) picked at (131.7398, 22.8524) picked at (86.6471, 20.4892) bodies 5 in component "GM67 + printer"
fillet "Fillet7" radius 10 2 edges at (53.5, 106.75, 100) (53.5, 106.75, 0) on bodies 5 in component "GM67 + printer"
fillet "Fillet8" radius 6 2 edges at (49.5, 76.75, 96) (49.5, 76.75, 4) on bodies 5 in component "GM67 + printer"
sketch "Scanner  cutout" plane through (60.6628, 0, -35.0237) normal (0.866025, 0, -0.5) x (0, 1, 0) in component "GM67 + printer"
  line L0 (0, 193.6025) -> (0, 162.2628) construction
  line L1 (0, 162.2628) -> (60, 162.2628) construction
  line L2 (60, 162.2628) -> (60, 193.6025) construction
  line L3 (60, 193.6025) -> (0, 193.6025) construction
  line L4 (0, 193.6025) -> (60, 193.6025) construction
  line L5 (0, 162.2628) -> (60, 162.2628) construction
  line L6 (60, 193.6025) -> (60, 162.2628) construction
  line L7 (0, 193.6025) -> (0, 162.2628) construction
  line L8 (30, 162.2628) -> (30, 193.6025) construction
  line L9 (44, 171.9327) -> (16, 171.9327)
  line L10 (16, 171.9327) -> (16, 183.9327)
  line L11 (16, 183.9327) -> (44, 183.9327)
  line L12 (44, 183.9327) -> (44, 171.9327)
  line L13 (44, 171.9327) -> (16, 183.9327) construction
  line L14 (16, 171.9327) -> (44, 183.9327) construction
  line L15 (43, 172.9327) -> (17, 172.9327)
  line L16 (17, 172.9327) -> (17, 182.9327)
  line L17 (17, 182.9327) -> (43, 182.9327)
  line L18 (43, 182.9327) -> (43, 172.9327)
  line L19 (16, 171.9327) -> (16, 170.1827)
  line L20 (16, 170.1827) -> (44, 170.1827)
  line L21 (44, 170.1827) -> (44, 171.9327)
  line L22 (0, 167.3327) -> (49, 167.3327)
  line L23 (49, 167.3327) -> (49, 163.3327)
  line L24 (49, 163.3327) -> (0, 163.3327)
  line L25 (0, 167.3327) -> (0, 163.3327)
  point P0 (30, 177.9327)
  dimension "d556" = 28
  dimension "d557" = 12
  dimension "d558" = 1
  dimension "d559" = 1.75
  dimension "d560" = 4
  dimension "d561" = 4.6
  dimension "d563" = 15.6699
  dimension "d564" = 15.6699
  dimension "d565" = 5
  dimension "d583" = 31.3397
  constraint coincident L0.start L3.end
  constraint coincident L2.end L3.start
  constraint coincident L0.end L1.start
  constraint coincident L1.end L2.start
  constraint midpoint L5 L8.start
  constraint midpoint L4 L8.end
  constraint horizontal L9
  constraint perpendicular L9 L10
  constraint parallel L9 L11
  constraint parallel L10 L12
  constraint coincident L13 P0
  constraint coincident L14 P0
  constraint coincident L8 P0
  constraint perpendicular L9 L19
  constraint perpendicular L19 L20
  constraint coincident L0 L22.start
  constraint perpendicular L7 L22
  constraint perpendicular L22 L23
  constraint coincident L7 L24.end
  constraint perpendicular L7 L24
  constraint collinear L12 L21
  measures "d556" distance of L10.end L11.end
  measures "d557" distance of L9.end L10.end
  measures "d559" distance of L9 L20
  measures "d560" distance of L22 L24
  measures "d561" distance of L9 L22
  measures "d563" distance of L4 P0
  measures "d564" distance of L5 P0
  measures "d565" distance of L12 L23
  measures "d583" distance of L4 L5
extrude "Extrude26" cut sketch "Printer Powersupply cutout" against normal up to surface (4 mm away) contours A0 | A1 picked at (30.1298, 39.1813) picked at (29.4986, 78.2625) bodies 5 in component "GM67 + printer"
extrude "Extrude27" add sketch "Printer Powersupply cutout" against normal blind 5 from surface at -4 contours L24 A2 L25 A3 | A4 | A5 picked at (22.8333, 64.9506) picked at (32.414, 77.9494) picked at (27.4278, 39.601) bodies 5 in component "GM67 + printer"
extrude "Extrude28" cut sketch "Power cutout (2)" against normal up to surface (4 mm away) contours A0 picked at (-22.2649, -31.183) bodies 5 in component "GM67 + printer"
extrude "Extrude29" cut sketch "Power cutout (2)" against normal blind 1.75 contours L10 L11 L12 L13 L14 L15 picked at (-27.9, -36.755) bodies 5 in component "GM67 + printer"
extrude "Extrude30" cut sketch "Printer Powersupply cutout" against normal up to surface (4 mm away) contours L37 A12 L38 A13 picked at (23.3333, 16.3333) bodies 5 in component "GM67 + printer"
extrude "Extrude31" add sketch "Base" along normal blind 4 from surface at 153.5 contours L5 L6 L7 A10 L22 picked at (1.3333, -134) bodies 5 in component "GM67 + printer"
fillet "Fillet9" radius 2 4 edges at (49.5, 20, 59.3) (49.5, 30, 29.75) (49.5, 40, 59.3) (49.5, 30, 88.85) on bodies 5 in component "GM67 + printer"
extrude "Extrude32" cut sketch "Printer Powersupply cutout" against normal blind 3.5 contours A4 | A5 picked at (32.414, 77.9494) picked at (27.4278, 39.601) bodies 5 in component "GM67 + printer"
extrude "Extrude33" add sketch "Printer Powersupply cutout" along normal blind 14.2 from surface at -49.5 contours A7 | A8 | A10 | A11 picked at (135.352, 15.8524) picked at (88.8813, 20.278) picked at (131.7398, 22.8524) picked at (86.6471, 20.4892) bodies 5 in component "GM67 + printer"
extrude "Extrude34" cut sketch "Printer Powersupply cutout" along normal up to surface (4 mm away) from surface at -53.5 contours A6 | A9 | A10 | A11 picked at (133.1154, 21.2809) picked at (84.1137, 21.38) picked at (131.7398, 22.8524) picked at (86.6471, 20.4892) bodies 5 in component "GM67 + printer"
fillet "Fillet10" radius 4 2 edges at (4, 128.156, 22.9197) (4, 78.156, 22.9197) on bodies 5 in component "GM67 + printer"
extrude "Extrude35" add sketch "Base" along normal up to surface (57.25 mm away) contours L8 L38 A36 | L8 A42 | L12 L38 A33 | L8 A5 L16 L17 L18 A14 A15 | L12 A17 | A6 S1 | A7 S0 picked at (54.3547, -10.8354) picked at (111.3605, -5.0148) picked at (54.3547, -89.1646) picked at (189.6849, -9.3579) picked at (111.3605, -94.9852) picked at (232.0947, -97.7086) picked at (161.4527, -131.5761) bodies 5 in component "GM67 + printer"
extrude "Extrude36" add sketch "Base" along normal up to surface (55.75 mm away) separate body contours A21 | A22 | A23 | A24 | A35 | A38 | A44 picked at (187.9895, -7.222) picked at (232.2154, -94.0645) picked at (118.8458, -94.7215) picked at (163.0278, -133.6914) picked at (56.0557, -91.0277) picked at (54.8223, -5.2785) picked at (115.2444, -6.2991) makes body 7 at (54.2551, 37.1667, 94.0456) makes body 8 at (236.3496, 37.1667, 92.8767) makes body 9 at (119.454, 37.1667, 93.9411) makes body 10 at (57.045, 37.1667, 4.6956) makes body 11 at (186.1518, 37.1667, 5.4217) makes body 12 at (167.1546, 37.1667, 132.8264) makes body 13 at (119.5786, 18.5833, 7.0525) in component "GM67 + printer"
extrude "Extrude42" add sketch "Base" along normal up to surface (81.25 mm away) from surface at 69.5 separate body contours L8 L37 L51 A48 | L12 L37 L43 A45 L52 picked at (48.6321, -7.7213) picked at (48.6321, -92.2787) makes body 14 at (45.3882, 123.6667, 4.6956) makes body 15 at (42.5983, 123.6667, 94.0456) in component "GM67 + printer"
extrude "Extrude43" add sketch "Base" along normal up to surface (77.25 mm away) from surface at 72 contours A20 | A41 | A47 | A50 picked at (8.9867, -6.9402) picked at (6.5557, -95.3155) picked at (44.3988, -91.0277) picked at (43.1655, -5.2785) bodies 14 15 makes body 16 at (4.7551, 123.5, 94.0456) makes body 17 at (9.0672, 123.5, 7.0525) in component "GM67 + printer"
extrude "Extrude44" add sketch "Base" along normal up to surface (153.5 mm away) contours A9 L13 L43 picked at (8.5199, -96.8371) bodies 15 17 16 5 14 in component "GM67 + printer"
sketch "Sketch1 (6)" plane through (0, 0, 0) normal (0, 0, 1) x (1, 0, 0) in component "Trial scanner"
  line L0 (-27.5, 15) -> (27.5, 15)
  line L1 (27.5, 15) -> (27.5, -15)
  line L2 (27.5, -15) -> (-27.5, -15)
  line L3 (-27.5, -15) -> (-27.5, 15)
  line L4 (-27.5, 15) -> (27.5, -15) construction
  line L5 (27.5, 15) -> (-27.5, -15) construction
  line L6 (23.5, -15) -> (23.5, 15)
  line L7 (23.5, 0) -> (22, 0)
  line L8 (22, 0) -> (-27.5, 0) construction
  line L9 (-16.15, 12.35) -> (10.25, 12.35) construction
  line L10 (10.25, 12.35) -> (10.25, -12.35) construction
  line L11 (10.25, -12.35) -> (-16.15, -12.35) construction
  line L12 (-16.15, -12.35) -> (-16.15, 12.35) construction
  line L13 (-16.15, 12.35) -> (10.25, -12.35) construction
  line L14 (10.25, 12.35) -> (-16.15, -12.35) construction
  circle A0 centre (10.25, -12.35) radius 1.25
  circle A1 centre (-16.15, -12.35) radius 1.25
  circle A2 centre (-16.15, 12.35) radius 1.25
  circle A3 centre (10.25, 12.35) radius 1.25
  circle A4 centre (10.25, -12.35) radius 2.5
  circle A5 centre (-16.15, -12.35) radius 2.5
  circle A6 centre (-16.15, 12.35) radius 2.5
  circle A7 centre (10.25, 12.35) radius 2.5
  point P0 (-2.95, 0)
  dimension "d526" = 55
  dimension "d527" = 30
  dimension "d528" = 4
  dimension "d533" = 26.4
  dimension "d534" = 24.7
  dimension "d535" = 2.5
  dimension "d536" = 5
  dimension "d550" = 13.25
  constraint horizontal L0
  constraint perpendicular L0 L1
  constraint parallel L0 L2
  constraint parallel L1 L3
  constraint coincident L4 origin
  constraint coincident L5 origin
  constraint coincident L2 L6.start
  constraint coincident L0 L6.end
  constraint perpendicular L0 L6
  constraint midpoint L6 L7.start
  constraint perpendicular L6 L7
  constraint midpoint L3 L8.end
  constraint horizontal L9
  constraint perpendicular L9 L10
  constraint parallel L9 L11
  constraint parallel L10 L12
  constraint coincident L13 P0
  constraint coincident L14 P0
  constraint coincident L8 P0
  constraint coincident L10.end L11.start
  constraint coincident L11.end L12.start
  constraint coincident L9.start L12.end
  constraint coincident L9.end L10.start
  constraint equal A0 A1
  constraint equal A1 A2
  constraint equal A2 A3
  constraint concentric A0 A4
  constraint concentric A1 A5
  constraint concentric A2 A6
  constraint concentric A3 A7
  constraint equal A4 A5
  constraint equal A5 A7
  constraint equal A6 A7
  measures "d526" distance of L1.end L2.end
  measures "d527" distance of L0.end L1.end
  measures "d528" distance of L1 L6
  measures "d533" distance of L10.end L11.end
  measures "d534" distance of L9.end L10.end
  measures "d535" diameter of A0
  measures "d536" diameter of A4
  measures "d550" distance of L6 L10
extrude "Extrude1'''''''" add sketch "Sketch1 (6)" along normal blind 20 separate body contours L0 L1 L2 L6 picked at (26.1667, 0) makes body 18 in component "Trial scanner"
extrude "Extrude2'''''" add sketch "Sketch1 (6)" against normal blind 4 contours L0 L2 L3 L6 | L0 L1 L2 L6 | A0 | A1 | A2 | A3 | A4 | A5 | A6 | A7 picked at (0.8391, 3.5499) picked at (26.1667, 0) picked at (10.5943, -12.5847) picked at (-15.7645, -12.7655) picked at (-15.7645, 11.9345) picked at (10.5943, 12.1153) picked at (12.3194, -12.5363) picked at (-14.0806, -12.5363) picked at (-14.0806, 12.1637) picked at (12.3194, 12.1637) bodies 18 in component "Trial scanner"
extrude "Extrude3'''''" cut sketch "Sketch1 (6)" against normal up to surface (4 mm away) contours A0 | A1 | A2 | A3 picked at (10.5943, -12.5847) picked at (-15.7645, -12.7655) picked at (-15.7645, 11.9345) picked at (10.5943, 12.1153) bodies 18 in component "Trial scanner"
extrude "Extrude4'''" add sketch "Sketch1 (6)" along normal blind 3 contours A4 | A5 | A6 | A7 picked at (12.3194, -12.5363) picked at (-14.0806, -12.5363) picked at (-14.0806, 12.1637) picked at (12.3194, 12.1637) bodies 18 in component "Trial scanner"
sketch "Sketch2 (3)" plane through (23.5, 0, 0) normal (-1, 0, 0) x (0, -1, 0) in component "Trial scanner"
  line L0 (-15, 0) -> (15, 0)
  line L1 (15, 0) -> (15, 20)
  line L2 (15, 20) -> (-15, 20)
  line L3 (-15, 20) -> (-15, 0)
  line L4 (0, 0) -> (0, 20) construction
  line L5 (14, 4.6) -> (-14, 4.6)
  line L6 (-14, 4.6) -> (-14, 16.6)
  line L7 (-14, 16.6) -> (14, 16.6)
  line L8 (14, 16.6) -> (14, 4.6)
  line L9 (14, 4.6) -> (-14, 16.6) construction
  line L10 (-14, 4.6) -> (14, 16.6) construction
  line L11 (15, 0) -> (-15, 0)
  line L12 (13, 5.6) -> (-13, 5.6)
  line L13 (-13, 5.6) -> (-13, 15.6)
  line L14 (-13, 15.6) -> (13, 15.6)
  line L15 (13, 15.6) -> (13, 5.6)
  line L16 (-14, 4.6) -> (-14, 2.85)
  line L17 (-14, 2.85) -> (14, 2.85)
  line L18 (14, 2.85) -> (14, 4.6)
  point P0 (0, 10.6)
  dimension "d541" = 28
  dimension "d542" = 12
  dimension "d544" = 4.6
  dimension "d545" = 1
  dimension "d553" = 1.75
  constraint coincident L4.start origin
  constraint midpoint L2 L4.end
  constraint horizontal L5
  constraint perpendicular L5 L6
  constraint parallel L5 L7
  constraint parallel L6 L8
  constraint coincident L9 P0
  constraint coincident L10 P0
  constraint coincident L4 P0
  constraint perpendicular L5 L16
  constraint perpendicular L16 L17
  measures "d541" distance of L6.end L7.end
  measures "d542" distance of L5.end L6.end
  measures "d544" distance of L5 L11
  measures "d553" distance of L5 L17
extrude "Extrude5'''" cut sketch "Sketch2 (3)" against normal up to surface (4 mm away) contours L12 L13 L14 L15 picked at (4.3333, 8.9333) bodies 18 in component "Trial scanner"
extrude "Extrude6''" cut sketch "Sketch2 (3)" against normal blind 3 contours L5 L6 L7 L8 picked at (4.3333, 4.9333) bodies 18 in component "Trial scanner"
fillet "Fillet1''" radius 10 2 edges at (-27.5, 15, -2) (-27.5, -15, -2) on bodies 18 in component "Trial scanner"
extrude "Extrude7'" cut sketch "Sketch2 (3)" against normal blind 2 contours L5 L16 L17 L18 picked at (4.6667, 3.4333) bodies 18 in component "Trial scanner"
extrude "Extrude45" cut sketch "Scanner  cutout" against normal up to surface (4 mm away) contours L15 L16 L17 L18 picked at (34.3333, 179.5993) bodies 5 15 17 14 16 in component "GM67 + printer"
extrude "Extrude46" cut sketch "Scanner  cutout" against normal blind 3 contours L9 L10 L11 L12 picked at (34.3333, 172.266) bodies 16 5 15 14 17 in component "GM67 + printer"
extrude "Extrude47" cut sketch "Scanner  cutout" against normal blind 2 contours L9 L19 L20 L21 picked at (34.6667, 171.3493) bodies 17 16 15 5 14 in component "GM67 + printer"
extrude "Extrude48" add sketch "Scanner  cutout" along normal blind 54 from surface at -4 contours L22 L23 L24 L25 picked at (16.3333, 165.9993) bodies 16 5 17 14 15 in component "GM67 + printer"